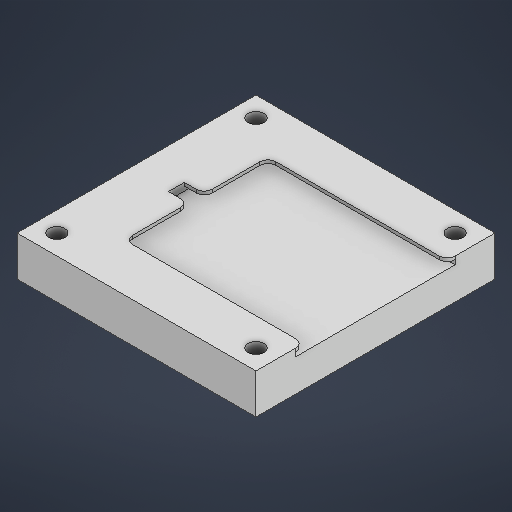
# Autodesk Inventor part: Flex Circuit Slot
Saved by Autodesk Inventor 2026.2 (Build 302298010, 298A)
## iProperties
Created: 2026-05-04
Part Number: Flex Circuit Slot
Material: Generic
Document SubType Name: Modeling
Designer: cfang
Density: 1 g/cm^3
Appearance: Default
Author: cfang
Autodesk Inventor part; units mm, degrees
ref_plane "YZ Plane" through (0, 0, 0) normal (1, 0, 0) x (0, 1, 0)
ref_plane "XZ Plane" through (0, 0, 0) normal (0, 1, 0) x (-1, 0, 0)
ref_plane "XY Plane" through (0, 0, 0) normal (0, 0, 1) x (1, 0, 0)
sketch "Sketch1" plane through (0, 0, 0) normal (0, 1, 0) x (-1, 0, 0)
  line L0 (-15, -15) -> (15, -15)
  line L1 (15, -15) -> (15, 15)
  line L2 (15, 15) -> (-15, 15)
  line L3 (-15, 15) -> (-15, -15)
  line L4 (-15, -15) -> (15, 15) construction
  line L5 (15, -15) -> (-15, 15) construction
  point P0 (0, 0)
  dimension "d0" = 30
  dimension "d1" = 30
  constraints: 12 end point, 2 midpoint, 2 parallel, 1 horizontal, 1 perpendicular
  measures "d0" distance of L0.end L1.end
  measures "d1" distance of L1.end L2.end
extrude "Extrusion1" add sketch "Sketch1" along normal blind 5
sketch "Sketch2" plane through (15, 0, 15) normal (1, 0, 0) x (0, 0, -1)
  line L0 (0, 5) -> (30, 5) projected
  line L1 (5, 4.05) -> (25, 4.05)
  line L2 (0, 0) -> (30, 0) projected
  line L3 (5, 4.6) -> (5, 4.05)
  line L4 (5, 4.6) -> (6, 4.6)
  line L5 (6, 4.6) -> (6, 5)
  line L6 (15, -1.7486) -> (15, 8.5822)
  line L7 (25, 4.05) -> (5, 4.05)
  line L8 (25, 4.6) -> (25, 4.05)
  line L9 (25, 4.6) -> (24, 4.6)
  line L10 (24, 4.6) -> (24, 5)
  point P0 (15, 0)
  point P1 (15, 0)
  point P2 (15, 0)
  dimension "d4" = 10
  dimension "d5" = 20
  dimension "d10" = 0.55
  dimension "d12" = 0.4
  dimension "d13" = 1
  constraints: 18 end point, 5 symmetric about line, 2 horizontal, 2 midpoint, 2 point on line, 1 perpendicular, 1 vertical
  measures "d4" horizontal distance of L1.start point (15, 0)
  measures "d5" distance of L1.start L1.end
  measures "d10" distance of L3.start L1.start
  measures "d12" distance of L4.end L5.end
  measures "d13" distance between parallel lines of L3 L5
extrude "Extrusion2" cut sketch "Sketch2" against normal blind 25
sketch "Sketch3" plane through (0, 5, 0) normal (0, 1, 0) x (1, 0, 0)
  line L0 (-10, 9) -> (15, 9) projected
  line L1 (15, -9) -> (-10, -9) projected
  line L2 (-10, 9) -> (-7.5, 9)
  line L3 (-7.5, 9) -> (-7.5, -9)
  line L4 (-7.5, -9) -> (-10, -9)
  line L5 (-10, -9) -> (-10, 9)
  line L6 (-7.5, -1) -> (-10, -1)
  line L7 (-10, -1) -> (-10, 1)
  line L8 (-10, 1) -> (-7.5, 1)
  line L9 (-7.5, 1) -> (-7.5, -1)
  point P0 (0, 0)
  dimension "d16" = 2.5
  dimension "d17" = 2
  dimension "d18" = 1
  constraints: 16 end point, 4 parallel, 3 point on line, 2 horizontal, 2 perpendicular
  measures "d16" distance between parallel lines of L5 L3
  measures "d17" distance between parallel lines of L6 L8
  measures "d18" distance from line of point (0, 0) L6
extrude "Extrusion3" add sketch "Sketch3" against normal up to surface (0.4 mm away) contours L0 L3 L8 L5 | L6 L3 L1 L5
fillet "Fillet1" radius 1 6 edges at (15, 4.8, 9) (15, 4.8, -9) (-7.5, 4.8, -1) (-7.5, 4.8, 1) (-7.5, 4.8, 9) (-7.5, 4.8, -9)
sketch "Sketch4" plane through (0, 5, 0) normal (0, 1, 0) x (1, 0, 0)
  point P0 (0, 0)
  point P1 (12.5, -12.5)
  point P2 (-12.5, -12.5)
  point P3 (-12.5, 12.5)
  point P4 (12.5, 12.5)
  dimension "d22" = 25
  dimension "d23" = 12.5
  dimension "d24" = 25
  dimension "d25" = 12.5
  constraints: 2 horizontal alignment, 2 vertical alignment
  measures "d22" distance of point (-12.5, -12.5) point (-12.5, 12.5)
  measures "d23" horizontal distance of point (-12.5, -12.5) point (0, 0)
  measures "d24" distance of point (12.5, -12.5) point (-12.5, -12.5)
  measures "d25" horizontal distance of point (-12.5, -12.5) point (0, 0)
hole "Hole1" at (12.5, 5, 12.5) at (-12.5, 5, 12.5) at (-12.5, 5, -12.5) at (12.5, 5, -12.5) direction (0, -1, 0) diameter 2 end through all
equation "\"d23\" = 0.5 * d22"
equation "\"d25\" = 0.5 * d24"
body "Solid1"
